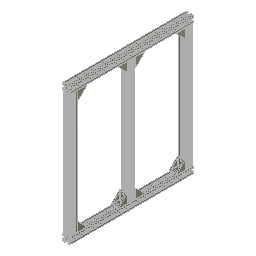
сборка станка вер 1.0(собрана рама станины) (Autodesk Fusion 360 design; units mm, degrees)
Autodesk Fusion 360 part; units mm, degrees
sketch "Sketch1" plane through (0, 0, 0) normal (0, 1, 0) x (1, 0, 0)
  line L0 (6.0101, -7) -> (-6.0101, -7)
  line L1 (-8.1, -12.8) -> (-8.1, -9.0899)
  line L2 (-6.0101, -7) -> (-8.1, -9.0899)
  line L3 (-4.1, -14.2) -> (-4.9, -14.2)
  line L4 (-4.9, -14.2) -> (-4.9, -15)
  line L5 (-4.1, -14.2) -> (-4.1, -12.8)
  line L6 (-13, -15) -> (-4.9, -15)
  line L7 (-8.1, -12.8) -> (-4.1, -12.8)
  line L8 (6.0101, -7) -> (8.1, -9.0899)
  line L9 (8.1, -12.8) -> (8.1, -9.0899)
  line L10 (8.1, -12.8) -> (4.1, -12.8)
  line L11 (4.1, -14.2) -> (4.1, -12.8)
  line L12 (4.1, -14.2) -> (4.9, -14.2)
  line L13 (4.9, -14.2) -> (4.9, -15)
  line L14 (13, -15) -> (4.9, -15)
  line L15 (14.2, -4.1) -> (14.2, -4.9)
  line L16 (12.8, -8.1) -> (9.0899, -8.1)
  line L17 (15, -13) -> (15, -4.9)
  line L18 (7, 6.0101) -> (9.0899, 8.1)
  line L19 (7, 6.0101) -> (7, -6.0101)
  line L20 (14.2, 4.9) -> (15, 4.9)
  line L21 (7, -6.0101) -> (9.0899, -8.1)
  line L22 (14.2, -4.1) -> (12.8, -4.1)
  line L23 (14.2, 4.1) -> (12.8, 4.1)
  line L24 (15, 13) -> (15, 4.9)
  line L25 (14.2, -4.9) -> (15, -4.9)
  line L26 (12.8, 8.1) -> (9.0899, 8.1)
  line L27 (12.8, 8.1) -> (12.8, 4.1)
  line L28 (12.8, -8.1) -> (12.8, -4.1)
  line L29 (14.2, 4.1) -> (14.2, 4.9)
  line L30 (4.1, 14.2) -> (4.9, 14.2)
  line L31 (8.1, 12.8) -> (8.1, 9.0899)
  line L32 (13, 15) -> (4.9, 15)
  line L33 (-6.0101, 7) -> (-8.1, 9.0899)
  line L34 (-6.0101, 7) -> (6.0101, 7)
  line L35 (-4.9, 14.2) -> (-4.9, 15)
  line L36 (6.0101, 7) -> (8.1, 9.0899)
  line L37 (4.1, 14.2) -> (4.1, 12.8)
  line L38 (-4.1, 14.2) -> (-4.1, 12.8)
  line L39 (-13, 15) -> (-4.9, 15)
  line L40 (4.9, 14.2) -> (4.9, 15)
  line L41 (-8.1, 12.8) -> (-8.1, 9.0899)
  line L42 (-8.1, 12.8) -> (-4.1, 12.8)
  line L43 (8.1, 12.8) -> (4.1, 12.8)
  line L44 (-4.1, 14.2) -> (-4.9, 14.2)
  line L45 (-14.2, 4.1) -> (-14.2, 4.9)
  line L46 (-12.8, 8.1) -> (-9.0899, 8.1)
  line L47 (-15, 13) -> (-15, 4.9)
  line L48 (-7, -6.0101) -> (-9.0899, -8.1)
  line L49 (-7, -6.0101) -> (-7, 6.0101)
  line L50 (-14.2, -4.9) -> (-15, -4.9)
  line L51 (-7, 6.0101) -> (-9.0899, 8.1)
  line L52 (-14.2, 4.1) -> (-12.8, 4.1)
  line L53 (-14.2, -4.1) -> (-12.8, -4.1)
  line L54 (-15, -13) -> (-15, -4.9)
  line L55 (-14.2, 4.9) -> (-15, 4.9)
  line L56 (-12.8, -8.1) -> (-9.0899, -8.1)
  line L57 (-12.8, -8.1) -> (-12.8, -4.1)
  line L58 (-12.8, 8.1) -> (-12.8, 4.1)
  line L59 (-14.2, -4.1) -> (-14.2, -4.9)
  circle A0 centre (0, 0) radius 5
  circle A1 centre (-11.55, -11.55) radius 2.25
  circle A2 centre (11.55, -11.55) radius 2.25
  circle A3 centre (11.55, 11.55) radius 2.25
  circle A4 centre (-11.55, 11.55) radius 2.25
  arc A5 (-15, -13) -> (-13, -15) centre (-13, -13) ccw
  arc A6 (13, -15) -> (15, -13) centre (13, -13) ccw
  arc A7 (15, 13) -> (13, 15) centre (13, 13) ccw
  arc A8 (-13, 15) -> (-15, 13) centre (-13, 13) ccw
  dimension "d17" = 10
  dimension "d22" = 4.5
  dimension "d24" = 360
  dimension "d25" = 2
  constraint coincident A0.centre origin
  constraint tangent L54 A5
  constraint tangent L6 A5
  constraint tangent L14 A6
  constraint tangent L17 A6
  constraint equal A5 A6
  constraint tangent L24 A7
  constraint tangent L32 A7
  constraint equal A5 A7
  constraint tangent L39 A8
  constraint tangent L47 A8
  constraint equal A5 A8
  measures "d17" diameter of A0
  measures "d22" diameter of A1
  measures "d25" radius of A5
extrude "Extrude1" add sketch "Sketch1" along normal blind 500 makes body 1
sketch "Sketch3" plane through (15, 0, 0) normal (1, 0, 0) x (0, 1, 0)
  line L0 (0, 13) -> (0, 4.9)
  line L1 (0, 4.9) -> (500, 4.9)
  line L2 (500, 4.9) -> (500, 13)
  line L3 (500, 13) -> (0, 13)
  line L4 (0, 15) -> (35, 15)
  line L5 (35, 15) -> (35, 19)
  line L6 (4, 50) -> (0, 50)
  line L7 (0, 50) -> (0, 15)
  line L8 (4, 50) -> (35, 19)
  line L9 (4, 50) -> (4, 19)
  line L10 (35, 19) -> (4, 19)
  dimension "d35" = 35
  dimension "d36" = 35
  dimension "d38" = 4
  dimension "d39" = 4
  dimension "d40" = 4
  constraint horizontal L4
  constraint vertical L5
  constraint horizontal L6
  constraint vertical L7
  constraint perpendicular L4 L9
  constraint perpendicular L9 L10
  measures "d35" distance of L4.start L4.end
  measures "d36" distance of L4.start L6.end
  measures "d38" distance of L6.end L6.start
  measures "d39" distance of L4.end L5.end
  measures "d40" distance of L7 L9
extrude "Extrude2" add sketch "Sketch3" against normal blind 30 separate body contours L4 L5 L6 L7 L9 L10 makes body 2
extrude "Extrude3" add sketch "Sketch3" against normal blind 4 contours L8 L9 L10 bodies 2 1
extrude "Extrude4" add sketch "Sketch3" along normal blind -26 and the other way blind 30 contours L8 L9 L10 bodies 1 2
sketch "Sketch4" plane through (0, 0, 19) normal (0, 0, 1) x (-1, 0, 0)
  line L0 (11, -35) -> (11, -4)
  line L1 (11, -4) -> (-11, -4)
  line L2 (-11, -4) -> (-11, -35)
  line L3 (-11, -35) -> (11, -35)
  line L4 (-11, -4) -> (-9, -4)
  circle A0 centre (0, -12.25) radius 3
  circle A1 centre (0, -27.25) radius 3
  point P0 (0, -35)
  dimension "d51" = 6
  dimension "d52" = 6
  constraint coincident L1.end L2.start
  constraint coincident L1 L4.end
  measures "d51" diameter of A0
  measures "d52" diameter of A1
extrude "Extrude5" cut sketch "Sketch4" against normal blind 8 contours A0 | A1 bodies 2 1
sketch "Sketch5" plane through (0, 4, 0) normal (0, 1, 0) x (-1, 0, 0)
  line L0 (11, 19) -> (11, 50)
  line L1 (11, 50) -> (-11, 50)
  line L2 (-11, 50) -> (-11, 19)
  line L3 (-11, 19) -> (11, 19)
  circle A0 centre (0, 41.75) radius 3
  circle A1 centre (0, 26.75) radius 3
  dimension "d57" = 6
  dimension "d58" = 6
  measures "d57" diameter of A0
  measures "d58" diameter of A1
extrude "Extrude6" cut sketch "Sketch5" against normal blind 6 contours A0 | A1 bodies 2
fillet "Fillet1" radius 3 1 edges at (0, 4, 19) on bodies 2
fillet "Fillet2" radius 2 6 edges at (11, 4, 36) (11, 4.8787, 19.8787) (11, 21, 19) (-11, 21, 19) (-11, 4.8787, 19.8787) (-11, 4, 36) on bodies 2
copy_body "Body->Comp1" bodies 2 removing the originals makes body 3 in component "уголок 30 2хМ6"
copy_body "Body->Comp2" bodies 1 removing the originals makes body 4 in component "профиль 3030 500mm"
move_body "Move1" bodies 3 to x (1, 0, 0) y (0, 1, 0) z (0, 0, 1) at (0, 30, 0) in component "уголок 30 2хМ6"
component "уголок 30 2хМ6" placed x (1, 0, 0) y (0, 1, 0) z (0, 0, 1) at (0, 0, 0)
component "профиль 3030 500mm" placed x (1, 0, 0) y (0, 1, 0) z (0, 0, 1) at (0, 0, 0)
component "профиль 3030 500mm" placed x (1, 0, 0) y (0, 0, -1) z (0, 1, 0) at (0, 485, 515)
component "профиль 3030 500mm" placed x (1, 0, 0) y (0, 0, -1) z (0, 1, 0) at (0, 15, 515)
component "профиль 3030 500mm" placed x (1, 0, 0) y (0, 0, -1) z (0, 1, 0) at (0, 235, 515)
component "уголок 30 2хМ6" placed x (1, 0, 0) y (0, 0, -1) z (0, 1, 0) at (0, 15.0029, 544.249)
component "уголок 30 2хМ6" placed x (1, 0, 0) y (0, 0, -1) z (0, 1, 0) at (0, 250.0029, 544.249)
component "уголок 30 2хМ6" placed x (1, 0, 0) y (0, 1, 0) z (0, 0, 1) at (0, 235, 0)
component "уголок 30 2хМ6" placed x (1, 0, 0) y (0, 0, 1) z (0, -1, 0) at (0, 249.249, -15.0029)
component "уголок 30 2хМ6" placed x (1, 0, 0) y (0, -1, 0) z (0, 0, -1) at (0, 264.252, 529.2461)
component "уголок 30 2хМ6" placed x (1, 0, 0) y (0, -1, 0) z (0, 0, -1) at (0, 499.252, 529.2461)
component "уголок 30 2хМ6" placed x (1, 0, 0) y (0, 0, 1) z (0, -1, 0) at (0, 484.249, -15.0029)
component "профиль 3030 500mm" placed x (1, 0, 0) y (0, 1, 0) z (0, 0, 1) at (0, 0, 530)
